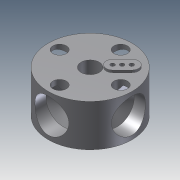
# Autodesk Inventor part: feed_wheel_rev4
Saved by Autodesk Inventor 2011 (Build 150239000, 239)
## iProperties
Created: 2012-11-10
Part Number: feed_wheel_rev4
Material: Default
Document SubType Name: Modeling
Designer: Administrator
Density: 1 g/cm^3
CQTools_X: 0
CQTools_Y: 0
CQTools_Z: 0
SweepLength: 0
Author: Administrator
Autodesk Inventor part; units mm, degrees
ref_plane "YZ Plane" through (0, 0, 0) normal (1, 0, 0) x (0, 1, 0)
ref_plane "XY Plane" through (0, 0, 0) normal (0, 0, 1) x (1, 0, 0)
sketch "Sketch2" plane through (0, 0, 0) normal (0, 0, 1) x (1, 0, 0)
  circle A0 centre (0, 0) radius 18.5
  circle A1 centre (0, 13.5) radius 3
  circle A2 centre (-13.5, 0) radius 3
  circle A3 centre (0, -13.5) radius 3
  circle A4 centre (13.5, 0) radius 3
  dimension "d2" = 37
  dimension "d90" = 6
  dimension "d93" = 360
  dimension "d95" = 2
  constraints: 5 centre point, 1 coincident, 1 vertical alignment, 9 other
  measures "d2" diameter of A0
  measures "d90" diameter of A1
extrude "wheel" add sketch "Sketch2" along normal mid plane 18.5 contours A0 | A1 | A2 | A3 | A4
sketch "Sketch4" plane through (0, 0, -9.25) normal (0, 0, -1) x (-1, 0, 0)
  circle A0 centre (0, 0) radius 18.5 projected
  line L0 (0, 0) -> (-13.0815, 13.0815) construction
  line L1 (0, 0) -> (0, 18.5) construction
  point P0 (-7.0711, 7.0711)
  dimension "d16" = 45
  dimension "d17" = 10
  constraints: 4 end point, 2 point on circle, 1 point on line, 1 vertical
  measures "d16" angle of L1 L0
  measures "d17" distance of L0.start point (-7.071, 7.071)
hole "servo mount hole" at (7.0711, 7.0711, -9.25) direction (0, 0, 1) diameter 2.2 depth 15
pattern_circular "servo mount pattern" count 4 over 360 about axis through (0, 0, 0) along (0, 0, 1) of "servo mount hole"
hole "center install hole" at (0, 0, -9.25) direction (0, 0, 1) diameter 8 end through all
sketch "Sketch6" plane through (0, 0, 9.25) normal (0, 0, 1) x (1, 0, 0)
  circle A0 centre (0, 0) radius 4 projected
  circle A1 centre (0, 0) radius 18.5 projected
  circle A2 centre (7.0711, 7.0711) radius 1.1 projected
  line L0 (0, 0) -> (2.8284, 2.8284) construction
  line L1 (7.0711, 7.0711) -> (13.0815, 13.0815) construction
  line L2 (2.8284, 2.8284) -> (7.0711, 7.0711) construction
  line L3 (4.9497, 4.9497) -> (9.1924, 9.1924) construction
  line L4 (7.0711, 7.0711) -> (11.3137, 11.3137) construction
  point P0 (4.9497, 4.9497)
  dimension "d37" = 6
  dimension "d40" = 3
  constraints: 10 end point, 3 collinear, 1 midpoint, 12 other
  measures "d37" distance of L0.end L1.start
  measures "d40" distance of point (4.95, 4.95) point (7.071, 7.071)
hole "shake wire holes" at (4.9497, 4.9497, 9.25) at (7.0711, 7.0711, 9.25) at (9.1924, 9.1924, 9.25) direction (0, 0, -1) diameter 1.82 depth 15
ref_plane "item hole plane" through (0, 18.5, 0) normal (0, 1, 0) x (-1, 0, 0)
sketch "Sketch8" plane through (0, 18.5, 0) normal (0, 1, 0) x (-1, 0, 0)
  point P0 (0, 0)
  point P1 (0, 0)
  constraints: 1 coincident
hole "item hole" at (0, 18.5, 0) direction (0, -1, 0) diameter 15 depth 6.5 tip angle 118
pattern_circular "item hole patterm" count 4 over 360 about axis through (0, 0, 0) along (0, 0, 1) of "item hole"
sketch "Sketch9" plane through (0, 0, 9.25) normal (0, 0, 1) x (1, 0, 0)
  circle A0 centre (9.1924, 9.1924) radius 0.91 projected
  circle A1 centre (7.0711, 7.0711) radius 0.91 projected
  circle A2 centre (4.9497, 4.9497) radius 0.91 projected
  circle A3 centre (4.9497, 4.9497) radius 2.91 construction
  line L0 (4.9497, 4.9497) -> (7.0711, 7.0711) construction
  circle A4 centre (7.0711, 7.0711) radius 2.91 construction
  line L1 (7.0711, 7.0711) -> (9.1924, 9.1924) construction
  circle A5 centre (9.1924, 9.1924) radius 2.91 construction
  line L2 (9.1924, 9.1924) -> (11.3137, 11.3137) construction
  line L3 (5.0134, 5.0134) -> (2.9567, 7.0701) construction
  line L4 (2.9567, 7.0701) -> (7.1342, 11.2496)
  line L5 (7.1342, 11.2496) -> (9.1924, 9.1924) construction
  line L6 (7.0701, 2.9567) -> (11.2496, 7.1342)
  arc A6 (2.9567, 7.0701) -> (7.0701, 2.9567) centre (5.0139, 5.0139) ccw
  arc A7 (11.2496, 7.1342) -> (7.1342, 11.2496) centre (9.2551, 9.2551) ccw
  dimension "d66" = 2
  dimension "d69" = 3
  constraints: 14 end point, 5 point on circle, 2 centre point, 2 symmetric about line, 2 tangent, 1 coincident, 1 collinear, 1 perpendicular, 1 point on line, 19 other
  measures "d69" distance of L0.start L1.start
extrude "shake wire support" add sketch "Sketch9" along normal blind 1
extrude "looking holes" cut sketch "Sketch2" along normal up to surface (9.25 mm away) contours A1 | A2 | A3 | A4
equation "\"d2\" = wheel_diameter"
equation "\"d3\" = item_width + 2 * wall_thickness"
equation "\"d40\" = 0.5 * d37"
equation "\"d56\" = item_width"
equation "\"d61\" = item_depth"
equation "\"d55\" = 0.5 * wheel_diameter"
equation "\"item_width\" = 15"
equation "\"item_depth\" = 6.5"
equation "\"wall_thickness\" = 1.75"
equation "\"wheel_diameter\" = 37"
body "Solid2"
